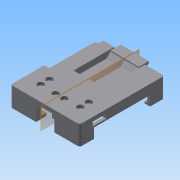
# Autodesk Inventor part: ZAPATO ZOWI DER2.1
Saved by Autodesk Inventor 2015 (Build 190159000, 159)
## iProperties
Created: 2015-06-30
Part Number: ZAPATO ZOWI DER2.1
Material: Generic
Document SubType Name: Modeling
Designer: pc
Density: 1 g/cm^3
Appearance: Default
Author: pc
Autodesk Inventor part; units mm, degrees
ref_plane "YZ Plane" through (0, 0, 0) normal (1, 0, 0) x (0, 1, 0)
ref_plane "XZ Plane" through (0, 0, 0) normal (0, 1, 0) x (-1, 0, 0)
ref_plane "XY Plane" through (0, 0, 0) normal (0, 0, 1) x (1, 0, 0)
sketch "Sketch2" plane through (0, 0, 0) normal (0, 1, 0) x (-1, 0, 0)
  line L0 (0, 0) -> (67.8, 0)
  line L1 (67.8, 0) -> (67.8, -19.2)
  line L2 (67.8, -19.2) -> (42.8, -19.2)
  line L3 (42.8, -19.2) -> (42.8, -16.2)
  line L4 (42.8, -16.2) -> (65, -16.2)
  line L5 (65, -16.2) -> (65, -8)
  line L6 (65, -8) -> (2.8, -8)
  line L7 (2.8, -8) -> (2.8, -16.2)
  line L8 (2.8, -16.2) -> (25, -16.2)
  line L9 (25, -16.2) -> (25, -19.2)
  line L10 (25, -19.2) -> (0, -19.2)
  line L11 (0, -19.2) -> (0, 0)
  dimension "d2" = 62.2
  dimension "d3" = 2.8
  dimension "d4" = 2.8
  dimension "d5" = 3
  dimension "d6" = 25
  dimension "d7" = 25
  dimension "d8" = 8
  dimension "d9" = 8.2
  constraints: 24 end point, 9 perpendicular, 4 point on line, 1 horizontal
  measures "d2" distance between parallel lines of L7 L5
  measures "d3" distance between parallel lines of L1 L5
  measures "d4" distance between parallel lines of L11 L7
  measures "d5" distance of L2.end L3.end
  measures "d6" distance of L1.end L2.end
  measures "d7" distance of L9.end L10.end
  measures "d8" distance between parallel lines of L0 L6
  measures "d9" distance between parallel lines of L6 L4
extrude "Extrusion1" add sketch "Sketch2" along normal blind 10
sketch "Sketch3" plane through (0, 0, 0) normal (0, -1, 0) x (1, 0, 0)
  line L0 (-2.8, -8) -> (-65, -8) projected
  line L1 (-42.8, -8) -> (-65, -8)
  line L2 (-65, -8) -> (-65, -16.2)
  line L3 (-65, -16.2) -> (-42.8, -16.2)
  line L4 (-42.8, -16.2) -> (-42.8, -8)
  line L5 (-42.8, -19.2) -> (-42.8, -16.2) projected
  line L6 (-42.8, -16.2) -> (-65, -16.2) projected
  line L7 (-25, -16.2) -> (-2.8, -16.2)
  line L8 (-2.8, -16.2) -> (-2.8, -8)
  line L9 (-2.8, -8) -> (-25, -8)
  line L10 (-25, -8) -> (-25, -16.2)
  line L11 (-65, -8) -> (-65, -16.2) projected
  point P0 (0, 0)
  constraints: 16 end point, 4 parallel, 3 collinear, 2 horizontal, 2 perpendicular, 1 point on line
extrude "Extrusion2" add sketch "Sketch3" against normal blind 5
sketch "Sketch7" plane through (0, 10, 0) normal (0, 1, 0) x (1, 0, 0)
  line L0 (0, 10) -> (0, 0)
  line L1 (0, 0) -> (-67.8, 0)
  line L2 (-67.8, 0) -> (-67.8, 19.2)
  line L3 (0, 10) -> (0, 19.2)
  line L4 (0, 19.2) -> (-2.8, 19.2)
  line L5 (-2.8, 19.2) -> (-2.8, 8)
  line L6 (-2.8, 8) -> (-65, 8)
  line L7 (-65, 8) -> (-65, 19.2)
  line L8 (-65, 19.2) -> (-67.8, 19.2)
  line L9 (-67.8, 19.2) -> (-67.8, 0) projected
  line L10 (0, 19.2) -> (-25, 19.2) projected
  line L11 (-2.8, 8) -> (-65, 8) projected
  line L12 (-65, 8) -> (-65, 16.2) projected
  line L13 (-2.8, 16.2) -> (-2.8, 8) projected
  constraints: 18 end point, 6 perpendicular, 5 collinear, 2 point on line, 2 vertical
extrude "Extrusion5" add sketch "Sketch7" along normal blind 73
sketch "Sketch10" plane through (0, 83, 0) normal (0, 1, 0) x (1, 0, 0)
  line L0 (-18.9, 0) -> (-48.9, 0)
  line L1 (-48.9, 0) -> (-48.9, 5)
  line L2 (-48.9, 5) -> (-18.9, 5)
  line L3 (-18.9, 5) -> (-18.9, 0)
  line L4 (-2.8, 8) -> (-65, 8) projected
  line L5 (-67.8, 0) -> (0, 0) projected
  line L6 (-33.9, 8) -> (-33.9, 19.521) construction
  line L7 (-33.9, 0) -> (-33.9, -9.399) construction
  dimension "d40" = 3
  dimension "d41" = 30
  constraints: 12 end point, 2 collinear, 2 midpoint, 2 parallel, 2 vertical, 1 horizontal, 1 perpendicular
  measures "d40" distance between parallel lines of L4 L2
  measures "d41" distance between parallel lines of L1 L3
extrude "Extrusion8" cut sketch "Sketch10" against normal blind 40
sketch "Sketch11" plane through (-48.9, 83, -5) normal (0, 0, 1) x (1, 0, 0)
  line L0 (0, 0) -> (1, 0)
  line L1 (1, 0) -> (1, -40)
  line L2 (1, -40) -> (0, -40)
  line L3 (0, -40) -> (0, 0)
  line L4 (29, 0) -> (30, 0)
  line L5 (30, 0) -> (30, -40)
  line L6 (30, -40) -> (29, -40)
  line L7 (29, -40) -> (29, 0)
  line L8 (30, -40) -> (0, -40) projected
  line L9 (30, 0) -> (30, -40) projected
  line L10 (0, -40) -> (0, 0) projected
  line L11 (0, 0) -> (30, 0) projected
  point P0 (48.9, -83)
  dimension "d44" = 1
  dimension "d45" = 1
  constraints: 16 end point, 4 collinear, 4 parallel, 2 horizontal, 2 perpendicular, 2 point on line
  measures "d44" distance between parallel lines of L3 L1
  measures "d45" distance between parallel lines of L5 L7
extrude "Extrusion9" cut sketch "Sketch11" against normal blind 30 contours L0 L1 L2 L3 | L4 L5 L6 L7
sketch "Sketch13" plane through (-2.8, 5, -8) normal (0, 0, -1) x (-1, 0, 0)
  line L0 (45.1, 78) -> (17.1, 78)
  line L1 (17.1, 78) -> (17.1, 73)
  line L2 (17.1, 73) -> (45.1, 73)
  line L3 (45.1, 73) -> (45.1, 78)
  line L4 (17.1, 78) -> (45.1, 78) projected
  line L5 (17.1, 78) -> (17.1, 38) projected
  line L6 (45.1, 38) -> (45.1, 78) projected
  point P0 (-2.8, -5)
  dimension "d48" = 5
  constraints: 8 end point, 3 collinear, 2 parallel, 1 horizontal, 1 perpendicular
  measures "d48" distance between parallel lines of L0 L2
extrude "Extrusion10" add sketch "Sketch13" along normal blind 3
chamfer "Chamfer1" distance 4 angle 45 1 edges at (-33.9, 83, -11)
fillet "Fillet1" radius 5 1 edges at (-33.9, 43, -5)
fillet "Fillet2" radius 2 4 edges at (0, 0, -9.6) (0, 83, -9.6) (-67.8, 0, -9.6) (-67.8, 83, -9.6)
sketch "Sketch16" plane through (-2.8, 5, -8) normal (0, 0, -1) x (-1, 0, 0)
  line L0 (65, 21.0579) -> (48, 21.0579)
  line L1 (48, 21.0579) -> (48, 7.5579)
  line L2 (48, 7.5579) -> (65, 7.5579)
  line L3 (65, 7.5579) -> (65, 21.0579)
  line L4 (24.35, 12) -> (37.85, 12)
  line L5 (37.85, 12) -> (37.85, -5)
  line L6 (37.85, -5) -> (24.35, -5)
  line L7 (24.35, -5) -> (24.35, 12)
  line L8 (40, -5) -> (22.2, -5) projected
  line L9 (22.2, -5) -> (22.2, 5) projected
  line L10 (62.2, 5) -> (62.2, 78) projected
  line L11 (65, -3) -> (65, 76) projected
  line L12 (-2.8, 21.0579) -> (14.2, 21.0579)
  line L13 (14.2, 21.0579) -> (14.2, 7.5579)
  line L14 (14.2, 7.5579) -> (-2.8, 7.5579)
  line L15 (-2.8, 7.5579) -> (-2.8, 21.0579)
  line L16 (-2.8, -3) -> (-2.8, 76) projected
  point P0 (-2.8, -5)
  dimension "d80" = 13.5
  dimension "d81" = 17
  dimension "d82" = 13.5
  dimension "d83" = 17
  dimension "d84" = 2.15
  dimension "d138" = 17
  constraints: 24 end point, 6 parallel, 5 collinear, 3 horizontal, 3 perpendicular
  measures "d80" distance of L2.end L0.start
  measures "d81" distance of L0.start L0.end
  measures "d82" distance of L4.start L4.end
  measures "d83" distance of L6.end L4.start
  measures "d84" distance between parallel lines of L7 L9
  measures "d138" distance of L12.start L12.end
extrude "Extrusion15" cut sketch "Sketch16" against normal blind 4
sketch "Sketch8" plane through (-25, 0, -8) normal (0, 0, -1) x (-1, 0, 0)
  circle A0 centre (4.65, 14.5) radius 1.25
  circle A1 centre (13.15, 14.5) radius 1.25
  line L0 (2.15, 17) -> (15.65, 17) projected
  line L1 (2.15, 0) -> (2.15, 17) projected
  line L2 (15.65, 17) -> (15.65, 0) projected
  circle A2 centre (28.3, 23.5579) radius 1.25
  circle A3 centre (28.3, 15.0579) radius 1.25
  line L3 (25.8, 26.0579) -> (40, 26.0579) projected
  line L4 (25.8, 12.5579) -> (25.8, 26.0579) projected
  line L5 (40, 12.5579) -> (25.8, 12.5579) projected
  circle A4 centre (-10.5, 23.5579) radius 1.25
  circle A5 centre (-10.5, 15.0579) radius 1.25
  line L6 (-8, 26.0579) -> (-8, 12.5579) projected
  line L7 (-8, 12.5579) -> (-25, 12.5579) projected
  line L8 (-25, 26.0579) -> (-8, 26.0579) projected
  point P0 (-25, 0)
  dimension "d28" = 2.5
  dimension "d29" = 2.5
  dimension "d87" = 2.5
  dimension "d88" = 2.5
  dimension "d89" = 2.5
  dimension "d90" = 2.5
  dimension "d91" = 2.5
  dimension "d92" = 2.5
  dimension "d93" = 2.5
  dimension "d94" = 2.5
  dimension "d95" = 2.5
  dimension "d96" = 2.5
  dimension "d139" = 2.5
  dimension "d140" = 2.5
  dimension "d141" = 2.5
  dimension "d142" = 2.5
  dimension "d143" = 2.5
  dimension "d144" = 2.5
  constraints: 6 centre point
  measures "d28" diameter of A1
  measures "d29" diameter of A0
  measures "d87" distance from line of L0 A0.centre
  measures "d88" distance from line of L1 A0.centre
  measures "d89" distance from line of L0 A1.centre
  measures "d90" distance from line of L2 A1.centre
  measures "d91" diameter of A2
  measures "d92" diameter of A3
  measures "d93" distance from line of L3 A2.centre
  measures "d94" distance from line of L4 A2.centre
  measures "d95" distance from line of L5 A3.centre
  measures "d96" distance from line of L4 A3.centre
  measures "d139" diameter of A4
  measures "d140" diameter of A5
  measures "d141" distance from line of L6 A5.centre
  measures "d142" distance from line of L7 A5.centre
  measures "d143" distance from line of L6 A4.centre
  measures "d144" distance from line of L8 A4.centre
extrude "Extrusion16" cut sketch "Sketch8" against normal up to surface (8 mm away)
sketch "Sketch15" plane through (-67.8, 0, 0) normal (0, 0, 1) x (1, 0, 0)
  circle A0 centre (53.3, 15.0579) radius 3
  circle A1 centre (53.3, 23.5579) radius 3
  circle A2 centre (38.15, 14.5) radius 3
  circle A3 centre (29.65, 14.5) radius 3
  circle A4 centre (14.5, 15.0579) radius 3
  circle A5 centre (14.5, 23.5579) radius 3
  circle A6 centre (53.3, 15.0579) radius 1.25 projected
  circle A7 centre (53.3, 23.5579) radius 1.25 projected
  circle A8 centre (38.15, 14.5) radius 1.25 projected
  circle A9 centre (29.65, 14.5) radius 1.25 projected
  circle A10 centre (14.5, 15.0579) radius 1.25 projected
  circle A11 centre (14.5, 23.5579) radius 1.25 projected
  point P0 (67.8, 0)
  dimension "d145" = 6
  dimension "d146" = 6
  dimension "d147" = 6
  dimension "d148" = 6
  dimension "d149" = 6
  dimension "d150" = 6
  constraints: 6 centre point, 6 concentric
  measures "d145" diameter of A0
  measures "d146" diameter of A1
  measures "d147" diameter of A2
  measures "d148" diameter of A3
  measures "d149" diameter of A4
  measures "d150" diameter of A5
extrude "Extrusion17" cut sketch "Sketch15" against normal blind 3
sketch "Sketch17" plane through (0, 83, 0) normal (0, 1, 0) x (1, 0, 0)
  line L0 (-65, 17.2) -> (-50, 17.2)
  line L1 (-50, 17.2) -> (-50, 19.2)
  line L2 (-50, 19.2) -> (-65, 19.2)
  line L3 (-65, 19.2) -> (-65, 17.2)
  line L4 (-65, 16.2) -> (-42.8, 16.2) projected
  line L5 (-65, 8) -> (-65, 19.2) projected
  line L6 (-42.8, 19.2) -> (-65, 19.2) projected
  point P0 (0, 0)
  dimension "d111" = 2
  dimension "d112" = 15
  constraints: 8 end point, 2 collinear, 2 parallel, 1 horizontal, 1 perpendicular
  measures "d111" distance of L0.end L1.end
  measures "d112" distance of L1.end L2.end
extrude "Extrusion18" add sketch "Sketch17" against normal blind 20
fillet "Fillet4" radius 2 1 edges at (-50, 83, -18.2)
sketch "Sketch18" plane through (0, 83, 0) normal (0, 1, 0) x (1, 0, 0)
  line L0 (-67.8, 0) -> (-59.8, 0)
  line L1 (-59.8, 0) -> (-59.8, 5)
  line L2 (-59.8, 5) -> (-67.8, 5)
  line L3 (-67.8, 5) -> (-67.8, 0)
  point P0 (0, 0)
  dimension "d116" = 8
  dimension "d117" = 5
  constraints: 8 end point, 2 parallel, 1 horizontal, 1 perpendicular
  measures "d116" distance of L0.start L0.end
  measures "d117" distance of L2.end L0.start
extrude "Extrusion19" cut sketch "Sketch18" against normal blind 50
sketch "Sketch19" plane through (0, 83, 0) normal (0, 1, 0) x (1, 0, 0)
  line L0 (-2.8, 19.2) -> (-5.3, 19.2)
  line L1 (-5.3, 19.2) -> (-5.3, 17.2)
  line L2 (-5.3, 17.2) -> (-2.8, 17.2)
  line L3 (-2.8, 17.2) -> (-2.8, 19.2)
  line L4 (-65, 17.2) -> (-52, 17.2) projected
  point P0 (0, 0)
  dimension "d120" = 2.5
  constraints: 8 end point, 2 parallel, 1 collinear, 1 horizontal, 1 perpendicular
  measures "d120" distance of L0.start L0.end
extrude "Extrusion20" add sketch "Sketch19" against normal up to surface (73 mm away)
sketch "Sketch20" plane through (0, 2, 0) normal (1, 0, 0) x (0, 0, -1)
  line L0 (19.2, 67) -> (9.5, 67)
  line L1 (9.5, 67) -> (9.5, 12)
  line L2 (9.5, 12) -> (19.2, 12)
  line L3 (19.2, 12) -> (19.2, 67)
  line L4 (19.2, 81) -> (0, 81) projected
  line L5 (0, -2) -> (19.2, -2) projected
  line L6 (19.2, 0) -> (19.2, 79) projected
  line L7 (8, 3) -> (8, 81) projected
  dimension "d123" = 14
  dimension "d124" = 14
  dimension "d126" = 1.5
  constraints: 8 end point, 2 parallel, 1 collinear, 1 horizontal, 1 perpendicular
  measures "d123" distance between parallel lines of L4 L0
  measures "d124" distance between parallel lines of L5 L2
  measures "d126" distance between parallel lines of L7 L1
extrude "Extrusion21" cut sketch "Sketch20" against normal blind 10
sketch "Sketch21" plane through (-47.9, 83, -5) normal (0, 0, 1) x (1, 0, 0)
  line L0 (28, -35) -> (28, 0) projected
  line L1 (0, -5) -> (28, -5)
  line L2 (28, -5) -> (28, 5)
  line L3 (28, 5) -> (0, 5)
  line L4 (0, 5) -> (0, -5)
  line L5 (0, 0) -> (0, -35) projected
  line L6 (0, -5) -> (28, -5) projected
  point P0 (47.9, -83)
  constraints: 8 end point, 3 collinear, 2 parallel, 1 horizontal, 1 perpendicular
extrude "Extrusion22" add sketch "Sketch21" along normal up to surface (5 mm away)
chamfer "Chamfer2" distance 4 angle 45 1 edges at (-33.9, 88, -5)
chamfer "Chamfer3" distance 4 angle 45 1 edges at (-33.9, 78, -5)
ref_plane "Work Plane2" through (-33.9, 2, 0) normal (1, 0, 0) x (0, 0, -1)
body "Solid1"
